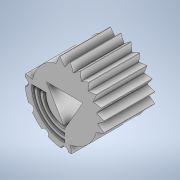
# Autodesk Inventor part: HandleGear
Saved by Autodesk Inventor 2021 (Build 250183000, 183)
## iProperties
Created: 2021-03-14
Part Number: HandleGear
Material: Generic
Document SubType Name: Modeling
Designer: ben
Density: 1 g/cm^3
Appearance: Default
Author: ben
Autodesk Inventor part; units mm, degrees
ref_plane "YZ Plane" through (0, 0, 0) normal (1, 0, 0) x (0, 1, 0)
ref_plane "XZ Plane" through (0, 0, 0) normal (0, 1, 0) x (-1, 0, 0)
ref_plane "XY Plane" through (0, 0, 0) normal (0, 0, 1) x (1, 0, 0)
sketch "Sketch1" plane through (0, 0, 0) normal (0, 0, 1) x (1, 0, 0)
  line L0 (12.4511, 7.2451) -> (-0.0489, -14.4055) projected
  line L1 (-0.0489, -14.4055) -> (-12.5489, 7.2451) projected
  line L2 (-12.5489, 7.2451) -> (12.4511, 7.2451) projected
  circle A0 centre (0, 0) radius 27.5 projected
  circle A1 centre (0, 0) radius 22.5
  line L3 (3.6703, 27.254) -> (6.9607, 19.2431)
  line L4 (6.9607, 19.2431) -> (-1.6221, 20.399)
  line L5 (-1.6221, 20.399) -> (3.6703, 27.254)
  line L6 (0, 27.5) -> (0, 14.4902)
  line L7 (-3.6703, 27.254) -> (-6.9607, 19.2431)
  line L8 (-6.9607, 19.2431) -> (1.6221, 20.399)
  line L9 (1.6221, 20.399) -> (-3.6703, 27.254)
  line L10 (3.7128, 20.1237) -> (10.5991, 25.3754)
  line L11 (10.5991, 25.3754) -> (11.704, 16.7859)
  line L12 (11.704, 16.7859) -> (3.7128, 20.1237)
  line L13 (8.7947, 18.4771) -> (16.8056, 21.7675)
  line L14 (16.8056, 21.7675) -> (15.6497, 13.1847)
  line L15 (15.6497, 13.1847) -> (8.7947, 18.4771)
  line L16 (13.2773, 15.5712) -> (21.8668, 16.6762)
  line L17 (21.8668, 16.6762) -> (18.5289, 8.685)
  line L18 (18.5289, 8.685) -> (13.2773, 15.5712)
  line L19 (16.855, 11.6043) -> (25.4378, 10.4484)
  line L20 (25.4378, 10.4484) -> (20.1454, 3.5934)
  line L21 (20.1454, 3.5934) -> (16.855, 11.6043)
  line L22 (19.2841, 6.8465) -> (27.2753, 3.5086)
  line L23 (27.2753, 3.5086) -> (20.389, -1.743)
  line L24 (20.389, -1.743) -> (19.2841, 6.8465)
  line L25 (20.399, 1.6221) -> (27.254, -3.6703)
  line L26 (27.254, -3.6703) -> (19.2431, -6.9607)
  line L27 (19.2431, -6.9607) -> (20.399, 1.6221)
  line L28 (0, 0) -> (-27.0822, 4.7753)
  line L29 (0, 0) -> (27.5, 0) construction
  line L30 (0, 0) -> (4.7753, -27.0822)
  line L31 (0, 0) -> (27.5, 0) construction
  circle A2 centre (-27.5, 0) radius 2.5
  circle A3 centre (-23.8157, -13.75) radius 2.5
  circle A4 centre (-13.75, -23.8157) radius 2.5
  circle A5 centre (0, -27.5) radius 2.5
  point P0 (0, 0)
  point P1 (3.003, 22.2987)
  point P2 (0, 22.5)
  point P3 (5.9522, 21.6984)
  point P4 (5.8234, 21.7333)
  point P5 (11.3654, 19.4185)
  point P6 (11.25, 19.4856)
  point P7 (16.004, 15.8153)
  point P8 (15.9099, 15.9099)
  point P9 (19.5519, 11.1343)
  point P10 (19.4856, 11.25)
  point P11 (21.7675, 5.6944)
  point P12 (21.7333, 5.8234)
  point P13 (22.4996, -0.1334)
  point P14 (22.5, 0)
  point P15 (21.6984, -5.9522)
  point P16 (21.6984, -5.9522)
  point P17 (22.5867, -0.067)
  point P18 (22.4996, -0.1334)
  point P19 (22.5, 0)
  point P20 (21.8345, 5.7812)
  point P21 (21.7675, 5.6944)
  point P22 (21.7333, 5.8234)
  point P23 (19.5942, 11.2354)
  point P24 (19.5519, 11.1343)
  point P25 (19.4856, 11.25)
  point P26 (16.0186, 15.9239)
  point P27 (16.004, 15.8153)
  point P28 (15.9099, 15.9099)
  point P29 (11.3514, 19.5272)
  point P30 (11.3654, 19.4185)
  point P31 (11.25, 19.4856)
  point P32 (5.9106, 21.7998)
  point P33 (5.8234, 21.7333)
  point P34 (0, 22.5)
  point P35 (0, 22.5)
  point P36 (-5.9522, 21.6984)
  point P37 (-2.4974, -27.3864)
  point P38 (2.4974, -27.3864)
  point P39 (3.9071, -22.1582)
  point P40 (-22.1582, 3.9071)
  point P41 (-27.3864, 2.4974)
  point P42 (-27.3864, -2.4974)
  point P43 (-24.966, -11.5304)
  point P44 (-22.4686, -15.856)
  point P45 (-15.856, -22.4686)
  point P46 (-11.5304, -24.966)
  dimension "d0" = 5
  dimension "d5" = 90
  dimension "d7" = 170
  dimension "d8" = 80
  dimension "d9" = 5
  dimension "d12" = 90
  constraints: 58 end point, 15 point on line, 7 point on circle, 5 centre point, 3 symmetric about line, 2 equal length, 2 horizontal, 2 vertical, 63 other
  measures "d0" radial gap between concentric circles of A0 A1
  measures "d7" angle of L29 L28
  measures "d8" angle of L30 L31
  measures "d9" diameter of A2
extrude "Extrusion1" add sketch "Sketch1" along normal blind 35 contours L2 L1 L28 A1 L7 L8 L4 L12 L15 L18 L21 L24 L27 L26 L30 L0 | L30 A1 L28 L1 L0 | L30 A0 A5 A4 A3 A2 L28 A1 | L26 L27 L24 L23 A1 | A1 L23 L25 L26 | L7 L9 A1 | A1 L5 L4 L8 L7 | L23 L24 L27 L25 A1 | A1 L25 L23 | L5 L3 L10 A1 | L6 L4 L5 | L9 L8 L6 | A1 L10 L12 L4 L8 L9 | L25 L27 L24 L21 L20 A1 | A1 L20 L22 L23 L25 | L10 L3 A1 | A1 L3 L4 L12 L10 | L20 L21 L24 L22 A1 | A1 L22 L20 | L21 L18 L17 A1 L22 L24 | L3 L10 L11 L13 A1 | A1 L13 L15 L12 L4 L3 | A1 L17 L19 L20 L22 | L21 L19 A1 L17 L18 | L18 L15 L14 A1 L19 L21 | L13 L11 A1 | A1 L11 L12 L15 L13 | L14 L16 A1 L11 L13 | L12 L11 A1 L16 L18 L15 | A1 L19 L17 | L17 L19 A1 L14 L16 | L18 L16 A1 L14 L15 | L14 A1 L16
sketch "Sketch2" plane through (0, 0, 35) normal (0, 0, 1) x (1, 0, 0)
  arc A0 (-14.9812, -0.75) -> (0, -15) centre (0, 0) ccw
  arc A1 (-16.9834, -0.75) -> (0, -17) centre (0, 0) ccw
  arc A2 (-18.9852, -0.75) -> (0, -19) centre (0, 0) ccw
  line L0 (0, 0) -> (0, -19) construction
  arc A3 (-20.9866, -0.75) -> (0, -21) centre (0, 0) ccw
  arc A4 (-22.9878, -0.75) -> (0, -23) centre (0, 0) ccw
  line L1 (-23, 0) -> (-22.9878, 0)
  line L2 (-13, 0) -> (-12.4416, 0)
  line L3 (-15, 0) -> (-16.75, 0)
  line L4 (-19.25, 0) -> (-20.75, 0)
  line L5 (0, -15) -> (0, -17)
  line L6 (0, -17) -> (0, -19)
  line L7 (0, -19) -> (0, -21)
  line L8 (0, -21) -> (0, -23)
  arc A5 (-20.75, 0) -> (-19.25, 0) centre (-20, 0) ccw
  arc A6 (-16.75, 0) -> (-15.25, 0) centre (-16, 0) ccw
  arc A7 (-13, 0) -> (0, -13) centre (0, 0) ccw
  line L9 (-14.9812, -0.75) -> (-14, -0.75)
  line L10 (-16.9834, -0.75) -> (-18, -0.75)
  line L11 (-18, -0.75) -> (-18.9852, -0.75)
  line L12 (-20.9866, -0.75) -> (-22, -0.75)
  line L13 (-22, -0.75) -> (-22.9878, -0.75)
  line L14 (-12.9783, -0.75) -> (-12.9783, 0.75)
  line L15 (-12.9783, 0.75) -> (-22.9878, 0.75)
  line L16 (-22.9878, 0.75) -> (-22.9878, -0.75)
  line L17 (-15.25, 0) -> (-14.9812, -0.75)
  line L18 (-16.75, 0) -> (-16.9834, -0.75)
  line L19 (-19.25, 0) -> (-18.9852, -0.75)
  line L20 (-20.75, 0) -> (-20.9866, -0.75)
  line L21 (-22.9878, -0.75) -> (-20.9866, -0.75)
  line L22 (-18.9852, -0.75) -> (-16.9834, -0.75)
  line L23 (-14.9812, -0.75) -> (-12.9783, -0.75)
  line L24 (0, 0) -> (-13, 0) construction
  line L25 (-15.25, 0) -> (-16.75, 0) construction
  line L26 (0, -15) -> (0, -13)
  circle A8 centre (-19.25, 0.75) radius 0.75
  circle A9 centre (-16.75, 0.75) radius 0.75
  point P0 (-12.9783, 0)
  dimension "d14" = 15
  dimension "d15" = 17
  dimension "d16" = 19
  dimension "d18" = 21
  dimension "d19" = 23
  dimension "d21" = 1.5
  dimension "d23" = 1.5
  dimension "d24" = 13
  dimension "d26" = 1.5
  dimension "d29" = 1.5
  dimension "d30" = 1.5
  constraints: 54 end point, 18 point on circle, 10 centre point, 8 collinear, 7 point on line, 6 coincident, 5 horizontal, 4 parallel, 3 perpendicular, 2 midpoint
  measures "d14" radius of A0
  measures "d15" radius of A1
  measures "d16" radius of A2
  measures "d18" radius of A3
  measures "d19" radius of A4
  measures "d21" diameter of A5
  measures "d23" diameter of A6
  measures "d24" radius of A7
  measures "d26" distance of L14.end L14.start
  measures "d29" diameter of A8
  measures "d30" diameter of A9
extrude "Extrusion2" cut sketch "Sketch2" against normal blind 10 contours L9 L23 A7 L26 A0 | L17 L3 A9 L15 L14 L2 A7 L23 L9 | A6 L3 | L6 A2 L11 L10 A1 | A9 L15 | L18 L10 L11 L19 A8 L15 A9 | L8 A4 L13 L12 A3 | A8 L15 | A5 L4 | L4 L20 L12 L13 L16 L15 A8 picked at (-16.8585, 0.4135) picked at (-19.3585, 0.4135)
fillet "Fillet1" radius 0.2 25 edges at (-3.6703, 27.254, 17.5) (-5.9522, 21.6984, 17.5) (0, 22.5, 17.5) (3.6703, 27.254, 17.5) (5.9106, 21.7998, 17.5) (10.5991, 25.3754, 17.5) (11.3514, 19.5272, 17.5) (16.8056, 21.7675, 17.5) (16.0186, 15.9239, 17.5) (21.8668, 16.6762, 17.5) (19.5942, 11.2354, 17.5) (25.4378, 10.4484, 17.5) (21.8345, 5.7812, 17.5) (27.2753, 3.5086, 17.5) (22.5867, -0.067, 17.5) (27.254, -3.6703, 17.5) (21.6984, -5.9522, 17.5) (2.4974, -27.3864, 17.5) (-2.4974, -27.3864, 17.5) (-15.856, -22.4686, 17.5) (-11.5304, -24.966, 17.5) (-24.966, -11.5304, 17.5) (-22.4686, -15.856, 17.5) (-27.3864, 2.4974, 17.5) (-27.3864, -2.4974, 17.5)
fillet "Fillet2" radius 0.1 4 edges at (-15.25, 0, 30) (-16.75, 0, 30) (-19.25, 0, 30) (-20.75, 0, 30)
body "Solid1"
